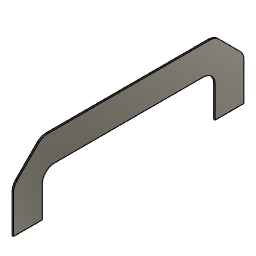
Side frame v4 (Autodesk Fusion 360 design; units mm, degrees)
Autodesk Fusion 360 part; units mm, degrees
sketch "Sketch1" plane through (0, 0, 0) normal (1, 0, 0) x (0, 1, 0)
  line L0 (180, 75) -> (-180, 75)
  line L1 (-240, 15) -> (-240, -75)
  line L2 (240, -75) -> (240, 15)
  line L3 (-240, -75) -> (-180, -75)
  line L4 (-180, -75) -> (-180, 75)
  line L5 (-240, 15) -> (-240, -75)
  line L6 (240, -75) -> (180, -75)
  line L7 (180, -75) -> (180, 75)
  line L8 (240, 15) -> (240, -75)
  line L9 (-180, 75) -> (180, 75)
  line L10 (240, 15) -> (-240, 15)
  line L11 (-240, 15) -> (-180, 75)
  line L12 (240, 15) -> (180, 75)
  line L13 (-240, -75) -> (-180, -75)
  line L14 (180, -75) -> (240, -75)
  line L15 (194.2857, 60.7143) -> (48, 15) construction
  line L16 (-194.2857, 60.7143) -> (-48, 15) construction
  line L17 (180, -56.25) -> (240, -75) construction
  line L18 (0, 55) -> (5, 55)
  line L19 (5, 35) -> (0, 35)
  line L20 (5, 65) -> (10, 65)
  line L21 (10, 65) -> (10, 25)
  line L22 (10, 25) -> (5, 25)
  line L23 (0, 75) -> (0, 55)
  line L24 (0, 35) -> (0, 15)
  line L25 (5, 25) -> (5, 35)
  line L26 (5, 55) -> (5, 65)
  dimension "d1" = 480
  dimension "d3" = 60
  dimension "d5" = 60
  constraint horizontal L0
  constraint perpendicular L0 L1
  constraint parallel L0 L13
  constraint parallel L1 L2
  constraint coincident origin L15
  constraint coincident origin L16
  constraint horizontal L3
  constraint vertical L4
  constraint vertical L5
  constraint horizontal L6
  constraint vertical L7
  constraint vertical L8
  constraint horizontal L9
  constraint horizontal L10
  constraint coincident L12 L15.start
  constraint coincident L11 L16.start
  constraint collinear L13 L14
  constraint coincident L7 L17.start
  constraint collinear L16 L17
  constraint coincident L10 L16.end
  constraint coincident L10 L15.end
  constraint midpoint L0 L23.start
  constraint midpoint L10 L24.end
  constraint horizontal L18
  constraint horizontal L19
  constraint horizontal L20
  constraint vertical L21
  constraint horizontal L22
  constraint vertical L25
  constraint collinear L23 L24
  constraint collinear L25 L26
  measures "d1" distance of L1.end L2.start
  measures "d3" distance of L1.end L3.end
  measures "d5" distance of L2.start L6.end
extrude "Extrude1" add sketch "Sketch1" along normal blind 3
sketch "Sketch2" plane through (0, 0, 0) normal (-1, 0, 0) x (0, -1, 0)
  line L0 (-180, -75) -> (-180, 15)
  line L1 (-180, 15) -> (180, 15)
  line L2 (180, 15) -> (180, -75)
  line L3 (180, -75) -> (240, -75)
  line L4 (240, -75) -> (240, 15)
  line L5 (240, 15) -> (180, 75)
  line L6 (180, 75) -> (-180, 75)
  line L7 (-180, 75) -> (-240, 15)
  line L8 (-240, 15) -> (-240, -75)
  line L9 (-240, -75) -> (-180, -75)
  line L10 (0, 55) -> (5, 55)
  line L11 (5, 35) -> (0, 35)
  line L12 (5, 65) -> (10, 65)
  line L13 (10, 65) -> (10, 25)
  line L14 (10, 25) -> (5, 25)
  line L15 (5, 25) -> (5, 35)
  line L16 (5, 55) -> (5, 65)
  line L17 (0, 55) -> (0, 75)
  line L18 (0, 35) -> (0, 15)
  constraint horizontal L10
  constraint horizontal L11
  constraint horizontal L12
  constraint vertical L13
  constraint horizontal L14
  constraint vertical L15
  constraint collinear L15 L16
  constraint midpoint L6 L17.end
  constraint perpendicular L10 L17
  constraint midpoint L1 L18.end
  constraint perpendicular L1 L18
fillet "Fillet1" radius 25 2 edges at (1.5, -180, 15) (1.5, 180, 15)
fillet "Fillet2" radius 25 4 edges at (1.5, -240, 15) (1.5, -180, 75) (1.5, 180, 75) (1.5, 240, 15)
sketch "Sketch3" plane through (3, 0, 0) normal (1, 0, 0) x (0, 1, 0)
  arc A0 (240, 4.6447) -> (232.6777, 22.3223) centre (215, 4.6447) ccw
  line L0 (232.6777, 22.3223) -> (187.3223, 67.6777)
  arc A1 (187.3223, 67.6777) -> (169.6447, 75) centre (169.6447, 50) ccw
  line L1 (169.6447, 75) -> (-169.6447, 75)
  arc A2 (-169.6447, 75) -> (-187.3223, 67.6777) centre (-169.6447, 50) ccw
  line L2 (-187.3223, 67.6777) -> (-232.6777, 22.3223)
  arc A3 (-232.6777, 22.3223) -> (-240, 4.6447) centre (-215, 4.6447) ccw
  line L3 (-240, 4.6447) -> (-240, -75)
  line L4 (-240, -75) -> (-180, -75)
  line L5 (-180, -75) -> (-180, -10)
  arc A4 (-155, 15) -> (-180, -10) centre (-155, -10) ccw
  line L6 (-155, 15) -> (155, 15)
  arc A5 (180, -10) -> (155, 15) centre (155, -10) ccw
  line L7 (180, -10) -> (180, -75)
  line L8 (180, -75) -> (240, -75)
  line L9 (240, -75) -> (240, 4.6447)
